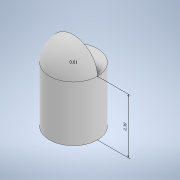
# Autodesk Inventor part: soft_1
Saved by Autodesk Inventor 2020 (Build 240168000, 168)
## iProperties
Created: 2020-01-22
Part Number: soft_1
Material: Generic
Document SubType Name: Modeling
Designer: sl65b
Density: 1 g/cm^3
Appearance: Default
Author: sl65b
Autodesk Inventor part; units mm, degrees
ref_plane "YZ Plane" through (0, 0, 0) normal (1, 0, 0) x (0, 1, 0)
ref_plane "XZ Plane" through (0, 0, 0) normal (0, 1, 0) x (-1, 0, 0)
ref_plane "XY Plane" through (0, 0, 0) normal (0, 0, 1) x (1, 0, 0)
sketch "Sketch1" plane through (0, 0, 0) normal (0, 0, 1) x (1, 0, 0)
  line L0 (0, 0) -> (-1, 0)
  line L1 (0, 0) -> (0, 2.3)
  line L2 (-1, 0.5) -> (-1, 2.3)
  line L3 (-1, 2.3) -> (0, 2.3)
  line L4 (-1, 0.5) -> (-1, 0)
  dimension "d10" = 2.3
  constraints: 10 end point, 2 perpendicular, 2 vertical, 1 horizontal
  measures "d10" distance of L0.start L1.end
revolve "Revolution1" add sketch "Sketch1" angle 360 about axis through (0, 0, 0) along (0, 1, 0)
sketch "Sketch2" plane through (0, 0, 0) normal (0, 0, 1) x (1, 0, 0)
  line L0 (1, 2.3) -> (-1, 2.3) projected
  line L1 (-1, 2.3) -> (0, 2.3)
  line L2 (0, 2.3) -> (0, 3.3)
  arc A0 (0, 3.3) -> (-1, 2.3) centre (0, 2.3) ccw
  point P0 (0, 0)
  dimension "d11" = 1
  dimension "d12" = 1
  constraints: 4 end point, 2 point on circle, 1 centre point, 1 horizontal, 1 midpoint, 1 vertical
  measures "d11" distance of L1.end L2.end
  measures "d12" radius of A0
revolve "Revolution3" add sketch "Sketch2" angle 180 about axis through (0, 2.3, 0) along (0, 1, 0)
sketch "Sketch4" plane through (0, 2.3, 0) normal (0, 1, 0) x (1, 0, 0)
  circle A0 centre (0, 0.01) radius 0.2492
  line L0 (1, 0) -> (-1, 0) projected
  point P0 (0, 0)
  dimension "d14" = 0.01
  constraints: 1 centre point
  measures "d14" distance from line of L0 A0.centre
body "Solid1"
